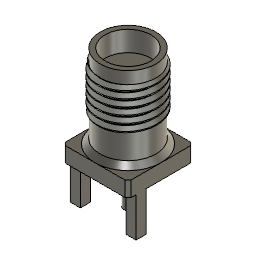
sma-female-straight-edgemount (Autodesk Fusion 360 design; units mm, degrees)
part number: 2026-08-08-15-43-03-547
Autodesk Fusion 360 part; units mm, degrees
sketch "Sketch1" plane through (0, 0, 0) normal (0, 0, 1) x (1, 0, 0)
  line L0 (3.25, 3.25) -> (-3.25, 3.25)
  line L1 (-3.25, 3.25) -> (-3.25, -3.25)
  line L2 (-3.25, -3.25) -> (3.25, -3.25)
  line L3 (3.25, -3.25) -> (3.25, 3.25)
  line L4 (3.25, 3.25) -> (-3.25, -3.25) construction
  line L5 (-3.25, 3.25) -> (3.25, -3.25) construction
  dimension "d1" = 6.5
  dimension "d2" = 6.5
  constraint horizontal L0
  constraint perpendicular L0 L1
  constraint parallel L0 L2
  constraint parallel L1 L3
  constraint coincident L4 origin
  constraint coincident L5 origin
  measures "d1" distance of L1.end L2.end
  measures "d2" distance of L0.end L1.end
extrude "Extrude1" add sketch "Sketch1" along normal blind 1.5
sketch "Sketch2" plane through (0, 0, 1.5) normal (0, 0, 1) x (-1, 0, 0)
  line L0 (-3.25, 3.25) -> (-3.25, -3.25)
  line L1 (-3.25, -3.25) -> (3.25, -3.25)
  line L2 (3.25, -3.25) -> (3.25, 3.25)
  line L3 (3.25, 3.25) -> (-3.25, 3.25)
  circle A0 centre (0, 0) radius 2.75
  dimension "d7" = 5.5
  constraint coincident A0.centre origin
  measures "d7" diameter of A0
extrude "Extrude2" add sketch "Sketch2" along normal blind 3 contours A0
sketch "Sketch3" plane through (0, 0, 4.5) normal (0, 0, 1) x (-1, 0, 0)
  circle A0 centre (0, 0) radius 2.75
  circle A1 centre (0, 0) radius 3.25
  dimension "d10" = 6.5
  constraint coincident A0.centre A1.centre
  measures "d10" diameter of A1
extrude "Extrude3" add sketch "Sketch3" along normal blind 4 contours A0 | A1
sketch "Sketch4" plane through (0, 0, 8.5) normal (0, 0, 1) x (-1, 0, 0)
  circle A0 centre (0, 0) radius 3.25
  circle A1 centre (0, 0) radius 2.75
  dimension "d13" = 5.5
  constraint coincident A0.centre A1.centre
  measures "d13" diameter of A1
extrude "Extrude4" add sketch "Sketch4" along normal blind 1 contours A1
extrude "Extrude5" add 1 faces at (-0.7525, -0.0891, 9.5) along direction (0, 0, 1) blind 0.2
sketch "Sketch5" plane through (0, 0, 0) normal (0, 0, -1) x (1, 0, 0)
  line L0 (3.25, -3.25) -> (3.25, 3.25)
  line L1 (3.25, 3.25) -> (-3.25, 3.25)
  line L2 (-3.25, 3.25) -> (-3.25, -3.25)
  line L3 (-3.25, -3.25) -> (3.25, -3.25)
  circle A0 centre (0, 0) radius 0.45
  line L4 (0, 0) -> (0, 0.45) construction
  line L5 (0, 0.45) -> (-3.25, 0.45) construction
  line L6 (0, 0.45) -> (3.25, 0.45) construction
  line L7 (3.25, 0.45) -> (3.25, 1.45) construction
  line L8 (3.25, 1.45) -> (-3.25, 1.45) construction
  line L9 (3.25, 1.45) -> (2.25, 1.45)
  line L10 (2.25, 1.45) -> (2.25, 2.45)
  line L11 (2.25, 2.45) -> (3.25, 2.45)
  line L12 (3.25, 2.45) -> (3.25, 1.45)
  line L13 (-3.25, 1.45) -> (-2.25, 1.45)
  line L14 (-2.25, 1.45) -> (-2.25, 2.45)
  line L15 (-2.25, 2.45) -> (-3.25, 2.45)
  line L16 (-3.25, 2.45) -> (-3.25, 1.45)
  dimension "d18" = 0.9
  dimension "d19" = 1
  dimension "d20" = 1
  dimension "d21" = 1
  dimension "d22" = 1
  dimension "d23" = 1
  constraint coincident A0.centre L4.start
  constraint coincident A0 L4.end
  constraint vertical L4
  constraint coincident L2 L5.end
  constraint tangent A0 L5
  constraint coincident L0 L6.end
  constraint tangent A0 L6
  constraint perpendicular L6 L7
  constraint coincident L2 L8.end
  constraint perpendicular L2 L8
  constraint horizontal L9
  constraint vertical L10
  constraint horizontal L11
  constraint vertical L12
  constraint horizontal L13
  constraint vertical L14
  constraint horizontal L15
  constraint vertical L16
  measures "d18" diameter of A0
  measures "d19" distance of L6.end L7.end
  measures "d20" distance of L7.end L9.end
  measures "d21" distance of L7.end L11.end
  measures "d22" distance of L8.end L13.end
  measures "d23" distance of L8.end L15.end
extrude "Extrude6" add sketch "Sketch5" along normal blind 4 contours L0 L9 L10 L11 L12 | L2 L13 L14 L15 L16 | A0
chamfer "Chamfer1" distance 0.3 angle 45 1 edges at (3.25, -3.25, 0.75) tangent chain off
chamfer "Chamfer2" distance 0.3 angle 45 3 edges at (-3.25, -3.25, 0.75) (-3.25, 3.25, 0.75) (3.25, 3.25, 0.75) tangent chain off
thread "Thread1" "ISO Metric profile 7.0 M7x0.5 M7x0.5 6g" major diameter 6.927 minor diameter 6.3505 pitch 0.5 angle 60 resizes the face on face at (-3.246, 0.162, 7.1667)
chamfer "Chamfer3" distance 0.1 angle 45 1 edges at (-0.4195, 0.1627, -4) tangent chain off
chamfer "Chamfer4" distance 0.1 angle 45 8 edges at (-2.75, -1.45, -4) (-3.25, -1.95, -4) (-2.75, -2.45, -4) (-2.25, -1.95, -4) (2.25, -1.95, -4) (2.75, -1.45, -4) (3.25, -1.95, -4) (2.75, -2.45, -4) tangent chain off
chamfer "Chamfer5" distance 0.5 angle 45 1 edges at (2.5639, -0.9944, 1.5) tangent chain off
sketch "Sketch6" plane through (0, 0, 9.7) normal (0, 0, 1) x (-1, 0, 0)
  circle A0 centre (0, 0) radius 2.75
  circle A1 centre (0, 0) radius 2.25
  dimension "d33" = 4.5
  constraint concentric A0 A1
  measures "d33" diameter of A1
extrude "Extrude7" cut sketch "Sketch6" against normal blind 2 contours A1
sketch "Sketch7" plane through (0, 0, 7.7) normal (0, 0, 1) x (-1, 0, 0)
  circle A0 centre (0, 0) radius 2.25
  circle A1 centre (0, 0) radius 0.45
  dimension "d36" = 0.9
  constraint coincident A0.centre A1.centre
  measures "d36" diameter of A1
extrude "Extrude8" cut sketch "Sketch7" against normal blind 1 contours A1
thread "Thread2" "ISO Metric profile 6.0 M6x0.7 M6x0.7 6g" major diameter 5.908 minor diameter 5.1087 pitch 0.7 angle 60 modelled right hand crest width 0.1005 on face at (-3.4463, 0.3449, 7.1667) crest through (-2.954, 0, 4.325)
